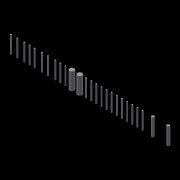
# Autodesk Inventor part: 3d_Welding_Tooling - Bot Wire
Saved by Autodesk Inventor 2018.3 (Build 223284000, 284)
## iProperties
Created: 2026-01-22
Part Number: 3d_Welding_Tooling - Bot Wire
Material: Genérico
Document SubType Name: Modeling
Designer: aca6
Density: 1 g/cm^3
Appearance: Valor por defecto
Author: aca6
Autodesk Inventor part; units mm, degrees
ref_plane "YZ Plane" through (0, 0, 0) normal (1, 0, 0) x (0, 1, 0)
ref_plane "XZ Plane" through (0, 0, 0) normal (0, 1, 0) x (-1, 0, 0)
ref_plane "XY Plane" through (0, 0, 0) normal (0, 0, 1) x (1, 0, 0)
sketch "Sketch1" plane through (0, 0, 0) normal (0, 0, 1) x (1, 0, 0)
  arc A0 (-20.8229, 0.5) -> (-20.8229, -0.5) centre (-22.5, 0) ccw
  line L0 (-19.6771, -0.5) -> (-20.8229, -0.5)
  arc A1 (-19.6771, -0.5) -> (-16.3229, -0.5) centre (-18, 0) ccw
  line L1 (-15.1771, -0.5) -> (-16.3229, -0.5)
  arc A2 (-15.1771, -0.5) -> (-11.8229, -0.5) centre (-13.5, 0) ccw
  line L2 (-10.6771, -0.5) -> (-11.8229, -0.5)
  arc A3 (-10.6771, -0.5) -> (-7.3229, -0.5) centre (-9, 0) ccw
  line L3 (-6.1771, -0.5) -> (-7.3229, -0.5)
  arc A4 (-6.1771, -0.5) -> (-2.8229, -0.5) centre (-4.5, 0) ccw
  line L4 (-1.6771, -0.5) -> (-2.8229, -0.5)
  arc A5 (-1.6771, -0.5) -> (1.6771, -0.5) centre (0, 0) ccw
  line L5 (2.8229, -0.5) -> (1.6771, -0.5)
  arc A6 (2.8229, -0.5) -> (6.1771, -0.5) centre (4.5, 0) ccw
  line L6 (7.3229, -0.5) -> (6.1771, -0.5)
  arc A7 (7.3229, -0.5) -> (10.6771, -0.5) centre (9, 0) ccw
  line L7 (11.8229, -0.5) -> (10.6771, -0.5)
  arc A8 (11.8229, -0.5) -> (15.1771, -0.5) centre (13.5, 0) ccw
  line L8 (16.3229, -0.5) -> (15.1771, -0.5)
  arc A9 (16.3229, -0.5) -> (19.6771, -0.5) centre (18, 0) ccw
  line L9 (20.8229, -0.5) -> (19.6771, -0.5)
  arc A10 (20.8229, -0.5) -> (20.8229, 0.5) centre (22.5, 0) ccw
  line L10 (19.6771, 0.5) -> (20.8229, 0.5)
  arc A11 (19.6771, 0.5) -> (16.3229, 0.5) centre (18, 0) ccw
  line L11 (15.1771, 0.5) -> (16.3229, 0.5)
  arc A12 (15.1771, 0.5) -> (11.8229, 0.5) centre (13.5, 0) ccw
  line L12 (10.6771, 0.5) -> (11.8229, 0.5)
  arc A13 (10.6771, 0.5) -> (7.3229, 0.5) centre (9, 0) ccw
  line L13 (6.1771, 0.5) -> (7.3229, 0.5)
  arc A14 (6.1771, 0.5) -> (2.8229, 0.5) centre (4.5, 0) ccw
  line L14 (1.6771, 0.5) -> (2.8229, 0.5)
  arc A15 (1.6771, 0.5) -> (-1.6771, 0.5) centre (0, 0) ccw
  line L15 (-2.8229, 0.5) -> (-1.6771, 0.5)
  arc A16 (-2.8229, 0.5) -> (-6.1771, 0.5) centre (-4.5, 0) ccw
  line L16 (-7.3229, 0.5) -> (-6.1771, 0.5)
  arc A17 (-7.3229, 0.5) -> (-10.6771, 0.5) centre (-9, 0) ccw
  line L17 (-11.8229, 0.5) -> (-10.6771, 0.5)
  arc A18 (-11.8229, 0.5) -> (-15.1771, 0.5) centre (-13.5, 0) ccw
  line L18 (-16.3229, 0.5) -> (-15.1771, 0.5)
  arc A19 (-16.3229, 0.5) -> (-19.6771, 0.5) centre (-18, 0) ccw
  line L19 (-20.8229, 0.5) -> (-19.6771, 0.5)
  line L20 (24.25, 0) -> (-24.25, 0) construction
  circle A20 centre (22.5, 0) radius 0.405
  circle A21 centre (18, 0) radius 0.405
  circle A22 centre (15, 0) radius 0.2025
  circle A23 centre (13.5, 0) radius 0.2025
  circle A24 centre (12, 0) radius 0.2025
  circle A25 centre (10.5, 0) radius 0.2025
  circle A26 centre (9, 0) radius 0.2025
  circle A27 centre (7.5, 0) radius 0.2025
  circle A28 centre (6, 0) radius 0.2025
  circle A29 centre (4.5, 0) radius 0.2025
  circle A30 centre (3, 0) radius 0.2025
  circle A31 centre (1.5, 0) radius 0.2025
  circle A32 centre (0, 0) radius 0.2025
  circle A33 centre (-1.5, 0) radius 0.2025
  circle A34 centre (-7.5, 0) radius 0.2025
  circle A35 centre (-9, 0) radius 0.2025
  circle A36 centre (-10.5, 0) radius 0.2025
  circle A37 centre (-12.6, 0) radius 0.2025
  circle A38 centre (-14.4, 0) radius 0.2025
  circle A39 centre (-16.5, 0) radius 0.2025
  circle A40 centre (-18, 0) radius 0.2025
  circle A41 centre (-19.5, 0) radius 0.2025
  circle A42 centre (-21.6, 0) radius 0.2025
  circle A43 centre (-23.4, 0) radius 0.2025
  line L21 (-25.25, -2) -> (-25.25, -0.4)
  arc A44 (-4.96, 0) -> (-6.33, 0) centre (-5.645, 0) ccw
  arc A45 (-6.33, 0) -> (-4.96, 0) centre (-5.645, 0) ccw
  arc A46 (-4.04, 0) -> (-2.67, 0) centre (-3.355, 0) ccw
  arc A47 (-2.67, 0) -> (-4.04, 0) centre (-3.355, 0) ccw
  point P0 (0, 0)
extrude "Extrusion1" add sketch "Sketch1" along normal blind 5 contours A20 | A21 | A22 | A23 | A24 | A25 | A26 | A27 | A28 | A29 | A30 | A31 | A32 | A33 | A34 | A35 | A36 | A37 | A38 | A39 | A40 | A41 | A42 | A43 | A45 A44 | A47 A46
body "Solid1"
